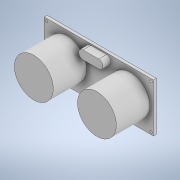
# Autodesk Inventor part: Ultrasonic HC-SRO4
Saved by Autodesk Inventor 2020 (Build 240168000, 168)
## iProperties
Created: 2021-04-26
Part Number: Ultrasonic HC-SRO4
Material: Типовые
Document SubType Name: Modeling
Designer: Антон
Density: 1 g/cm^3
Appearance: По умолчанию
Author: Антон
Autodesk Inventor part; units mm, degrees
ref_plane "YZ Plane" through (0, 0, 0) normal (1, 0, 0) x (0, 1, 0)
ref_plane "XZ Plane" through (0, 0, 0) normal (0, 1, 0) x (-1, 0, 0)
ref_plane "XY Plane" through (0, 0, 0) normal (0, 0, 1) x (1, 0, 0)
sketch "Эскиз1" plane through (0, 0, 0) normal (0, 0, 1) x (1, 0, 0)
  line L0 (0, 0) -> (45, 0)
  line L1 (45, 0) -> (45, 20)
  line L2 (45, 20) -> (0, 20)
  line L3 (0, 20) -> (0, 0)
  dimension "d0" = 45
  dimension "d1" = 20
  constraints: 8 end point, 2 parallel, 1 horizontal, 1 perpendicular
  measures "d0" distance of L2.end L1.end
  measures "d1" distance of L1.end L0.end
extrude "Выдавливание1" add sketch "Эскиз1" along normal blind 1.2
sketch "Эскиз2" plane through (0, 0, 1.2) normal (0, 0, 1) x (1, 0, 0)
  line L0 (0, 20) -> (0, 0) projected
  line L1 (0, 10) -> (1.5, 10)
  line L2 (1.5, 10) -> (9.5, 10)
  circle A0 centre (9.5, 10) radius 8
  line L3 (45, 20) -> (0, 20) projected
  line L4 (22.5, 20) -> (22.5, 0)
  line L5 (0, 0) -> (45, 0) projected
  circle A1 centre (35.5, 10) radius 8
  dimension "d5" = 16
  dimension "d4" = 1.5
  constraints: 6 end point, 3 midpoint, 2 horizontal, 1 centre point, 1 coincident, 1 horizontal alignment, 1 symmetric about line, 3 other
  measures "d4" distance of L1.start L1.end
extrude "Выдавливание2" add sketch "Эскиз2" along normal blind 13.8 contours A0 | A1
sketch "Эскиз3" plane through (0, 0, 1.2) normal (0, 0, 1) x (1, 0, 0)
  line L0 (45, 20) -> (0, 20) projected
  line L1 (22.5, 20) -> (22.5, 19.5)
  line L2 (27.5, 17.75) -> (17.5, 17.75) construction
  line L3 (25.75, 19.5) -> (19.25, 19.5)
  line L4 (19.25, 16) -> (25.75, 16)
  arc A0 (25.75, 16) -> (25.75, 19.5) centre (25.75, 17.75) ccw
  arc A1 (19.25, 19.5) -> (19.25, 16) centre (19.25, 17.75) ccw
  point P0 (0, 0)
  point P1 (22.5, 17.75)
  dimension "d8" = 0.5
  dimension "d9" = 10
  dimension "d10" = 3.5
  constraints: 10 end point, 6 point on circle, 4 tangent, 3 midpoint, 2 centre point, 2 point on line, 1 horizontal, 1 parallel, 1 vertical
  measures "d8" distance of L1.end L1.start
  measures "d9" distance of L2.start L2.end
  measures "d10" diameter of A1
extrude "Выдавливание3" add sketch "Эскиз3" along normal blind 3.3
sketch "Эскиз8" plane through (0, 0, 0) normal (0, 0, -1) x (-1, 0, 0)
  line L0 (-45, 0) -> (-45, 20) projected
  line L1 (-45, 20) -> (-44, 20)
  line L2 (-45, 20) -> (0, 20) projected
  line L3 (-44, 20) -> (-44, 19)
  circle A0 centre (-44, 19) radius 0.5
  line L4 (-45, 10) -> (0, 10)
  line L5 (0, 20) -> (0, 0) projected
  line L6 (-22.5, 20) -> (-22.5, 0)
  line L7 (0, 0) -> (-45, 0) projected
  circle A1 centre (-44, 1) radius 0.5
  circle A2 centre (-1, 19) radius 0.5
  circle A3 centre (-1, 1) radius 0.5
  dimension "d41" = 1
  dimension "d42" = 1
  dimension "d43" = 1
  constraints: 8 end point, 4 centre point, 4 midpoint, 3 symmetric about line, 1 coincident, 1 perpendicular, 1 point on line, 3 other
  measures "d41" distance of L0.end L1.end
  measures "d42" distance of L1.end L3.end
  measures "d43" diameter of A0
extrude "Выдавливание8" cut sketch "Эскиз8" against normal through all contours A0 | A1 | A2 | A3
sketch "Эскиз4" plane through (0, 0, 0) normal (0, 0, -1) x (-1, 0, 0)
  line L0 (-27.5, 2.5) -> (-17.5, 2.5)
  line L1 (-17.5, 2.5) -> (-17.5, 0)
  line L2 (-17.5, 0) -> (-27.5, 0)
  line L3 (-27.5, 0) -> (-27.5, 2.5)
  line L4 (-27.5, 2.5) -> (-17.5, 0) construction
  line L5 (-17.5, 2.5) -> (-27.5, 0) construction
  line L6 (0, 0) -> (-45, 0) projected
  point P0 (-22.5, 1.25)
  point P1 (-22.5, 0)
  dimension "d13" = 10
  dimension "d14" = 2.5
  constraints: 12 end point, 4 midpoint, 2 parallel, 1 horizontal, 1 perpendicular
  measures "d13" distance between parallel lines of L1 L3
  measures "d14" distance between parallel lines of L2 L0
extrude "Выдавливание4" add sketch "Эскиз4" along normal blind 3.3
sketch "Эскиз5" plane through (0, 0, -3.3) normal (0, 0, -1) x (-1, 0, 0)
  line L0 (-26.5, 1.5) -> (-26, 1.5)
  line L1 (-26, 1.5) -> (-26, 1)
  line L2 (-26, 1) -> (-26.5, 1)
  line L3 (-26.5, 1) -> (-26.5, 1.5)
  line L4 (-26.5, 1.25) -> (-27.5, 1.25)
  line L5 (-27.5, 2.5) -> (-27.5, 0) projected
  line L6 (-24, 1.5) -> (-23.5, 1.5)
  line L7 (-23.5, 1.5) -> (-23.5, 1)
  line L8 (-23.5, 1) -> (-24, 1)
  line L9 (-24, 1) -> (-24, 1.5)
  line L10 (-21.5, 1.5) -> (-21, 1.5)
  line L11 (-21, 1.5) -> (-21, 1)
  line L12 (-21, 1) -> (-21.5, 1)
  line L13 (-21.5, 1) -> (-21.5, 1.5)
  line L14 (-19, 1.5) -> (-18.5, 1.5)
  line L15 (-18.5, 1.5) -> (-18.5, 1)
  line L16 (-18.5, 1) -> (-19, 1)
  line L17 (-19, 1) -> (-19, 1.5)
  point P0 (0, 0)
  point P1 (-24, 1.25)
  point P2 (-21.5, 1.25)
  point P3 (-19, 1.25)
  dimension "d17" = 0.5
  dimension "d18" = 0.5
  dimension "d19" = 1
  dimension "d22" = 2.5
  constraints: 34 end point, 2 horizontal, 2 midpoint, 2 parallel, 2 perpendicular, 27 other
  measures "d17" distance of L1.end L2.end
  measures "d18" distance of L0.end L1.end
  measures "d19" distance of L4.start L4.end
  measures "d22" distance of L0.start L6.start
extrude "Выдавливание5" add sketch "Эскиз5" along normal blind 2
sketch "Эскиз6" plane through (26, 1, -3.3) normal (0, -1, 0) x (1, 0, 0)
  line L0 (0.5, -2) -> (0, -2) projected
  line L1 (0, 0) -> (0, -2) projected
  line L2 (0.5, -2) -> (0, -2)
  line L3 (0, -2) -> (0, -1.5)
  line L4 (0, -1.5) -> (0.5, -1.5)
  line L5 (0.5, -1.5) -> (0.5, -2)
  line L6 (-2, -2) -> (-2.5, -2)
  line L7 (-2.5, -2) -> (-2.5, -1.5)
  line L8 (-2.5, -1.5) -> (-2, -1.5)
  line L9 (-2, -1.5) -> (-2, -2)
  line L10 (-4.5, -2) -> (-5, -2)
  line L11 (-5, -2) -> (-5, -1.5)
  line L12 (-5, -1.5) -> (-4.5, -1.5)
  line L13 (-4.5, -1.5) -> (-4.5, -2)
  line L14 (-7, -2) -> (-7.5, -2)
  line L15 (-7.5, -2) -> (-7.5, -1.5)
  line L16 (-7.5, -1.5) -> (-7, -1.5)
  line L17 (-7, -1.5) -> (-7, -2)
  point P0 (-26, 3.3)
  dimension "d31" = 2.5
  constraints: 32 end point, 2 horizontal, 2 parallel, 2 perpendicular, 1 point on line, 24 other
  measures "d31" distance of L3.end L7.end
extrude "Выдавливание6" add sketch "Эскиз6" along normal blind 7
sketch "Эскиз7" plane through (0, 0, 1.2) normal (0, 0, 1) x (1, 0, 0)
  line L0 (26.5, 1.5) -> (26, 1.5) projected
  line L1 (26.5, 1) -> (26.5, 1.5) projected
  line L2 (26, 1.5) -> (26, 1) projected
  line L3 (26, 1) -> (26.5, 1) projected
  line L4 (21, 1) -> (21.5, 1) projected
  line L5 (21.5, 1) -> (21.5, 1.5) projected
  line L6 (21.5, 1.5) -> (21, 1.5) projected
  line L7 (21, 1.5) -> (21, 1) projected
  line L8 (26.5, 1.5) -> (26, 1.5) projected
  line L9 (26, 1.5) -> (26, 1) projected
  line L10 (26, 1) -> (26.5, 1) projected
  line L11 (26.5, 1) -> (26.5, 1.5) projected
  line L12 (23.5, 1) -> (24, 1) projected
  line L13 (24, 1) -> (24, 1.5) projected
  line L14 (24, 1.5) -> (23.5, 1.5) projected
  line L15 (23.5, 1.5) -> (23.5, 1) projected
  line L16 (18.5, 1) -> (19, 1) projected
  line L17 (19, 1) -> (19, 1.5) projected
  line L18 (19, 1.5) -> (18.5, 1.5) projected
  line L19 (18.5, 1.5) -> (18.5, 1) projected
  line L20 (17.5, 0) -> (17.5, 2.5) projected
  line L21 (17.5, 2.5) -> (27.5, 2.5) projected
  line L22 (27.5, 2.5) -> (27.5, 0) projected
  line L23 (27.5, 0) -> (17.5, 0) projected
  point P0 (0, 0)
extrude "Выдавливание7" add sketch "Эскиз7" along normal blind 1.8 contours L1 L3 L2 L0 | L7 L6 L5 L4 | L15 L14 L13 L12 | L19 L18 L17 L16
fillet "Сопряжение1" radius 0.5 16 edges at (21.25, 1.5, 1.2) (21.25, 1, 1.2) (21.5, 1.25, 1.2) (21, 1.25, 1.2) (18.75, 1, 1.2) (18.5, 1.25, 1.2) (19, 1.25, 1.2) (18.75, 1.5, 1.2) (23.75, 1, 1.2) (24, 1.25, 1.2) (23.5, 1.25, 1.2) (23.75, 1.5, 1.2) (26.25, 1.5, 1.2) (26, 1.25, 1.2) (26.25, 1, 1.2) (26.5, 1.25, 1.2)
